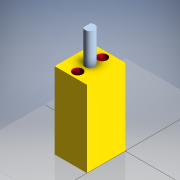
# Autodesk Inventor part: mini_motor
Saved by Autodesk Inventor 2016 (Build 200138000, 138)
## iProperties
Created: 2017-09-19
Part Number: mini_motor
Material: Wood (Cherry)
Document SubType Name: Modeling
Designer: student
Density: 0.63 g/cm^3
Appearance: Cherry - Natural Low Gloss
Author: student
Autodesk Inventor part; units mm, degrees
ref_plane "YZ Plane" through (0, 0, 0) normal (1, 0, 0) x (0, 1, 0)
ref_plane "XZ Plane" through (0, 0, 0) normal (0, 1, 0) x (-1, 0, 0)
ref_plane "XY Plane" through (0, 0, 0) normal (0, 0, 1) x (1, 0, 0)
sketch "Sketch1" plane through (0, 0, 0) normal (0, 1, 0) x (-1, 0, 0)
  line L0 (0, 0) -> (10.16, 0)
  line L1 (10.16, 0) -> (10.16, 12.065)
  line L2 (10.16, 12.065) -> (0, 12.065)
  line L3 (0, 12.065) -> (0, 0)
  dimension "d0" = 10.16
  dimension "d1" = 12.065
  constraints: 8 end point, 2 parallel, 1 horizontal, 1 perpendicular
  measures "d0" distance of L2.end L1.end
  measures "d1" distance of L1.end L0.end
extrude "Extrusion1" add sketch "Sketch1" along normal blind 24.13
sketch "Sketch2" plane through (0, 24.13, 0) normal (0, 1, 0) x (1, 0, 0)
  line L0 (0, 0) -> (-10.16, 0) construction
  line L1 (-10.16, 0) -> (-10.16, -12.065) construction
  line L2 (-10.16, -12.065) -> (0, -12.065) construction
  line L3 (0, -12.065) -> (0, 0) construction
  arc A0 (-6.096, -7.1684) -> (-6.096, -4.8966) centre (-5.08, -6.0325) ccw
  line L4 (-6.096, -4.8966) -> (-6.096, -7.1684)
  line L5 (-10.16, -12.065) -> (0, -12.065) construction
  line L6 (-5.08, -12.065) -> (-5.08, -9.906) construction
  circle A1 centre (-5.08, -9.906) radius 1.524
  circle A2 centre (-5.08, -6.0325) radius 2.2225 construction
  line L7 (0, -6.0325) -> (-10.16, -6.0325) construction
  line L8 (-10.16, 0) -> (-10.16, -12.065) construction
  circle A3 centre (-5.08, -2.159) radius 1.524
  dimension "d12" = 2.159
  dimension "d13" = 3.048
  dimension "d14" = 4.445
  constraints: 6 end point, 4 centre point, 3 midpoint, 2 coincident, 2 point on circle, 2 vertical, 1 symmetric about line, 1 other
  measures "d12" distance of L6.start L6.end
  measures "d13" diameter of A1
  measures "d14" diameter of A2
extrude "Extrusion2" add sketch "Sketch2" along normal blind 10.16 contours L4 A0
sketch "Sketch3" plane through (0, 24.13, 0) normal (0, 1, 0) x (1, 0, 0)
  circle A0 centre (-5.08, -9.906) radius 1.524 projected
  circle A1 centre (-5.08, -2.159) radius 1.524 projected
  point P0 (0, 0)
extrude "Extrusion3" cut sketch "Sketch3" against normal blind 3
body "Solid1"
